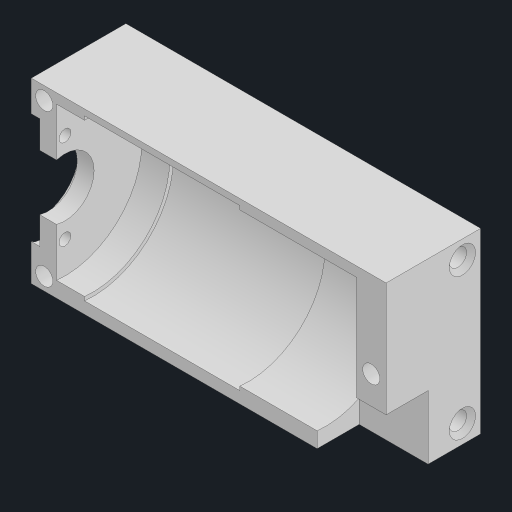
# Autodesk Inventor part: right_motor_holder
Saved by Autodesk Inventor 2023 (Build 270158000, 158)
## iProperties
Created: 2024-04-24
Part Number: right_motor_holder
Material: Generic
Document SubType Name: Modeling
Designer: szymo
Density: 1 g/cm^3
Appearance: Default
Author: szymo
Autodesk Inventor part; units mm, degrees
ref_plane "YZ Plane" through (0, 0, 0) normal (1, 0, 0) x (0, 1, 0)
ref_plane "XZ Plane" through (0, 0, 0) normal (0, 1, 0) x (-1, 0, 0)
ref_plane "XY Plane" through (0, 0, 0) normal (0, 0, 1) x (1, 0, 0)
ref_plane "Work Plane1" through (-42.7, -68.375, 15.375) normal (1, 0, 0) x (0, -1, 0)
sketch "Sketch1" plane through (-42.7, -68.375, 15.375) normal (1, 0, 0) x (0, -1, 0)
  circle A0 centre (0, 0) radius 14.375 projected
  circle A1 centre (0, 0) radius 13.7 projected
  line L0 (90.625, 18.375) -> (-15.375, 18.375) projected
  line L1 (-15.375, 18.375) -> (-15.375, 15.375) projected
  line L2 (90.625, 15.375) -> (-15.375, 15.375) projected
  line L3 (90.625, 18.375) -> (90.625, 15.375) projected
  line L4 (-15.375, 15.375) -> (16.375, 15.375)
  line L5 (16.375, 15.375) -> (16.375, -1.5)
  line L6 (16.375, -1.5) -> (-15.375, -1.5)
  line L7 (-15.375, -1.5) -> (-15.375, 15.375)
  circle A2 centre (0, 0) radius 13.9
  point P0 (-68.375, 15.375)
  point P1 (14.375, 0)
  point P2 (-13.6176, -1.5)
  point P3 (13.6176, -1.5)
  point P4 (16.375, 15.375)
  dimension "d1" = 2
  dimension "d2" = 1.5
  dimension "d3" = 0.2
  constraints: 8 end point, 2 parallel, 1 centre point, 1 horizontal, 1 horizontal alignment, 1 perpendicular, 2 other
  measures "d1" distance from line of L5 point (14.375, 0)
  measures "d2" distance from line of L6 point (14.375, 0)
  measures "d3" radial gap between concentric circles of A1 A2
extrude "Extrusion1" add sketch "Sketch1" along normal blind 9.5 contours A0 L6 A2 | A0 L6 L7 L2 L5 | A2 L6 A1 picked at (14.0681, 1.1841) picked at (-2.3687, 13.4988)
ref_plane "Work Plane2" through (-37.7, -68.375, 15.375) normal (1, 0, 0) x (0, -1, 0)
sketch "Sketch2" plane through (-37.7, -68.375, 15.375) normal (1, 0, 0) x (0, -1, 0)
  arc A0 (13.6176, -1.5) -> (-13.6176, -1.5) centre (0, 0) ccw projected
  line L0 (13.6176, -1.5) -> (16.375, -1.5) projected
  line L1 (16.375, -1.5) -> (16.375, 15.375) projected
  line L2 (16.375, 15.375) -> (-15.375, 15.375) projected
  line L3 (-15.375, 15.375) -> (-15.375, -1.5) projected
  line L4 (-15.375, -1.5) -> (-13.6176, -1.5) projected
  circle A1 centre (8, 0) radius 1.0564 projected
  circle A2 centre (-8, 0) radius 1.0564 projected
  circle A3 centre (0, 0) radius 5 projected
  circle A4 centre (0, 0) radius 13.7 projected
  circle A5 centre (0, 0) radius 5.2
  arc A6 (13.6176, -1.5) -> (-13.6176, -1.5) centre (0, 0) ccw projected
  line L5 (13.6176, -1.5) -> (-13.6176, -1.5)
  point P0 (-68.375, 15.375)
  point P1 (4.979, -1.5)
  point P2 (-4.979, -1.5)
  dimension "d6" = 0.2
  constraints: 2 end point, 1 centre point, 1 collinear
  measures "d6" radial gap between concentric circles of A3 A5
extrude "Extrusion2" add sketch "Sketch2" along normal blind 3 contours L5 A5 A0
sketch "Sketch3" plane through (-34.7, -68.375, 15.375) normal (1, 0, 0) x (0, 0, -1)
  arc A0 (-1.5, -13.6176) -> (-1.5, 13.6176) centre (0, 0) ccw projected
  line L0 (-1.5, 13.6176) -> (-1.5, 4.979) projected
  arc A1 (-1.5, -4.979) -> (-1.5, 4.979) centre (0, 0) ccw projected
  line L1 (-1.5, -4.979) -> (-1.5, -13.6176) projected
  circle A2 centre (0, -8) radius 1.0564 projected
  circle A3 centre (0, 8) radius 1.0564 projected
  arc A4 (0.512, -3.83) -> (1.6707, -5.5993) centre (4.9979, -2.1562) ccw projected
  arc A5 (1.6707, -5.5993) -> (2.5261, -5.269) centre (0, 0) ccw projected
  arc A6 (2.5261, -5.269) -> (2.195, -3.1802) centre (-2.2517, -4.9556) ccw projected
  arc A7 (2.195, -3.1802) -> (2.6654, -2.7976) centre (0, 0) ccw projected
  arc A8 (2.6654, -2.7976) -> (4.6428, -3.548) centre (5.3108, 1.1933) ccw projected
  arc A9 (4.6428, -3.548) -> (5.1407, -2.778) centre (0, 0) ccw projected
  arc A10 (5.1407, -2.778) -> (3.645, -1.2826) centre (1.0912, -5.3327) ccw projected
  arc A11 (3.645, -1.2826) -> (3.8008, -0.6966) centre (0, 0) ccw projected
  arc A12 (3.8008, -0.6966) -> (5.8416, -0.1414) centre (3.5951, 4.087) ccw projected
  arc A13 (5.8416, -0.1414) -> (5.7918, 0.7742) centre (0, 0) ccw projected
  arc A14 (5.7918, 0.7742) -> (3.7028, 1.1048) centre (4.0173, -3.6729) ccw projected
  arc A15 (3.7028, 1.1048) -> (3.4844, 1.6705) centre (0, 0) ccw projected
  arc A16 (3.4844, 1.6705) -> (4.809, 3.3192) centre (0.5063, 5.4196) ccw projected
  arc A17 (4.809, 3.3192) -> (4.2306, 4.0306) centre (0, 0) ccw projected
  arc A18 (4.2306, 4.0306) -> (2.3462, 3.0703) centre (5.4089, -0.6101) ccw projected
  arc A19 (2.3462, 3.0703) -> (1.8371, 3.3995) centre (0, 0) ccw projected
  arc A20 (1.8371, 3.3995) -> (1.9396, 5.512) centre (-2.776, 4.6821) ccw projected
  arc A21 (1.9396, 5.512) -> (1.0535, 5.7475) centre (0, 0) ccw projected
  arc A22 (1.0535, 5.7475) -> (0.0935, 3.863) centre (4.7345, 2.6857) ccw projected
  arc A23 (0.0935, 3.863) -> (-0.512, 3.83) centre (0, 0) ccw projected
  arc A24 (-0.512, 3.83) -> (-1.6707, 5.5993) centre (-4.9979, 2.1562) ccw projected
  arc A25 (-1.6707, 5.5993) -> (-2.5261, 5.269) centre (0, 0) ccw projected
  arc A26 (-2.5261, 5.269) -> (-2.195, 3.1802) centre (2.2517, 4.9556) ccw projected
  arc A27 (-2.195, 3.1802) -> (-2.6654, 2.7976) centre (0, 0) ccw projected
  arc A28 (-2.6654, 2.7976) -> (-4.6428, 3.548) centre (-5.3108, -1.1933) ccw projected
  arc A29 (-4.6428, 3.548) -> (-5.1407, 2.778) centre (0, 0) ccw projected
  arc A30 (-5.1407, 2.778) -> (-3.645, 1.2826) centre (-1.0912, 5.3327) ccw projected
  arc A31 (-3.645, 1.2826) -> (-3.8008, 0.6966) centre (0, 0) ccw projected
  arc A32 (-3.8008, 0.6966) -> (-5.8416, 0.1414) centre (-3.5951, -4.087) ccw projected
  arc A33 (-5.8416, 0.1414) -> (-5.7918, -0.7742) centre (0, 0) ccw projected
  arc A34 (-5.7918, -0.7742) -> (-3.7028, -1.1048) centre (-4.0173, 3.6729) ccw projected
  arc A35 (-3.7028, -1.1048) -> (-3.4844, -1.6705) centre (0, 0) ccw projected
  arc A36 (-3.4844, -1.6705) -> (-4.809, -3.3192) centre (-0.5063, -5.4196) ccw projected
  arc A37 (-4.809, -3.3192) -> (-4.2306, -4.0306) centre (0, 0) ccw projected
  arc A38 (-4.2306, -4.0306) -> (-2.3462, -3.0703) centre (-5.4089, 0.6101) ccw projected
  arc A39 (-2.3462, -3.0703) -> (-1.8371, -3.3995) centre (0, 0) ccw projected
  arc A40 (-1.8371, -3.3995) -> (-1.9396, -5.512) centre (2.776, -4.6821) ccw projected
  arc A41 (-1.9396, -5.512) -> (-1.0535, -5.7475) centre (0, 0) ccw projected
  arc A42 (-1.0535, -5.7475) -> (-0.0935, -3.863) centre (-4.7345, -2.6857) ccw projected
  arc A43 (-0.0935, -3.863) -> (0.512, -3.83) centre (0, 0) ccw projected
  circle A44 centre (0, 0) radius 7
  arc A45 (-1.5, -13.6176) -> (-1.5, 13.6176) centre (0, 0) ccw projected
  line L2 (-1.5, -13.6176) -> (-1.5, -16.375) projected
  line L3 (-1.5, -16.375) -> (15.375, -16.375) projected
  line L4 (15.375, -16.375) -> (15.375, 15.375) projected
  line L5 (15.375, 15.375) -> (-1.5, 15.375) projected
  line L6 (-1.5, 15.375) -> (-1.5, 13.6176) projected
  circle A46 centre (0, -8) radius 2.4
  circle A47 centre (0, 8) radius 2.4
  circle A48 centre (0, 0) radius 5.8433
  point P0 (15.375, 68.375)
  point P1 (2.019, 6.7025)
  point P2 (2.019, -6.7025)
  point P3 (-1.5, -9.8735)
  point P4 (-1.5, 9.8735)
  dimension "d9" = 14
  dimension "d10" = 4.8
  dimension "d11" = 4.8
  constraints: 4 centre point, 4 coincident, 1 concentric
  measures "d9" diameter of A44
  measures "d10" diameter of A46
  measures "d11" diameter of A47
extrude "Extrusion3" add sketch "Sketch3" along normal up to surface (1.5 mm away) contours L1 A46 A44 A47 L0 A0
sketch "Sketch4" plane through (-42.7, -84.75, 16.875) normal (0, 0, 1) x (1, 0, 0)
  line L0 (0, 2.7574) -> (0, 0) projected
  line L1 (0, 0) -> (9.5, 0) projected
  line L2 (9.5, 0) -> (9.5, 6.5015) projected
  line L3 (8, 6.5015) -> (9.5, 6.5015) projected
  line L4 (8, 11.396) -> (8, 6.5015) projected
  line L5 (5, 11.396) -> (8, 11.396) projected
  line L6 (5, 11.396) -> (5, 2.7574) projected
  line L7 (0, 2.7574) -> (5, 2.7574) projected
  line L8 (0, 31.75) -> (0, 29.9926) projected
  line L9 (0, 29.9926) -> (5, 29.9926) projected
  line L10 (5, 29.9926) -> (5, 21.354) projected
  line L11 (5, 21.354) -> (8, 21.354) projected
  line L12 (8, 26.2485) -> (8, 21.354) projected
  line L13 (8, 26.2485) -> (9.5, 26.2485) projected
  line L14 (9.5, 31.75) -> (9.5, 26.2485) projected
  line L15 (0, 31.75) -> (9.5, 31.75) projected
  circle A0 centre (7.2, 2.3) radius 2.5
  circle A1 centre (7.2, 29.45) radius 2.5
  point P0 (42.7, 84.75)
  dimension "d14" = 5
  dimension "d15" = 5
  dimension "d16" = 2.3
  dimension "d17" = 2.3
  dimension "d18" = 2.3
  dimension "d19" = 2.3
  constraints: 2 centre point, 2 coincident
  measures "d14" diameter of A0
  measures "d15" diameter of A1
  measures "d16" distance from line of A1.centre L14
  measures "d17" distance from line of A1.centre L15
  measures "d18" distance from line of L1 A0.centre
  measures "d19" distance from line of L2 A0.centre
hole "Hole1" at (-35.5, -82.45, 16.875) at (-35.5, -55.3, 16.875) direction (0, 0, -1) diameter 3.1 end through all clearance for "Countersunk Flat Head Screw ISO 2009/7046" size "M2.5" standard "ISO"
sketch "Sketch5" plane through (-42.7, -68.375, 15.375) normal (-1, 0, 0) x (0, 0, 1)
  circle A0 centre (0, 0) radius 14.375 projected
  arc A1 (1.5, 13.6176) -> (1.5, -13.6176) centre (0, 0) ccw projected
  line L0 (1.5, 15.375) -> (1.5, 13.6176) projected
  line L1 (-15.375, 15.375) -> (1.5, 15.375) projected
  line L2 (-15.375, -16.375) -> (-15.375, 15.375) projected
  line L3 (1.5, -16.375) -> (-15.375, -16.375) projected
  line L4 (1.5, -13.6176) -> (1.5, -16.375) projected
  point P0 (-15.375, 68.375)
  point P1 (1.5, -14.2965)
  point P2 (1.5, 14.2965)
ref_plane "Work Plane3" through (-70.4, -82.75, 1) normal (-1, 0, 0) x (0, 0, 1)
extrude "Extrusion4" add sketch "Sketch5" along normal up to surface (27.7 mm away) contours A0 L4 L3 L2 L1 L0
sketch "Sketch6" plane through (-70.4, -68.375, 15.375) normal (-1, 0, 0) x (0, 0, 1)
  line L0 (-15.375, 15.375) -> (1.5, 15.375) projected
  line L1 (-15.375, -16.375) -> (-15.375, 15.375) projected
  line L2 (1.5, -16.375) -> (-15.375, -16.375) projected
  line L3 (1.5, -14.2965) -> (1.5, -16.375) projected
  arc A0 (1.5, 14.2965) -> (1.5, -14.2965) centre (0, 0) ccw projected
  line L4 (1.5, 15.375) -> (1.5, 14.2965) projected
  circle A1 centre (0, 0) radius 13.7 projected
  line L5 (-15.375, 15.375) -> (1.5, 15.375)
  line L6 (1.5, 15.375) -> (1.5, -16.375)
  line L7 (1.5, -16.375) -> (-15.375, -16.375)
  line L8 (-15.375, -16.375) -> (-15.375, 15.375)
  point P0 (-15.375, 68.375)
  point P1 (1.5, 14.2965)
  point P2 (1.5, -14.2965)
  point P3 (1.5, -13.6176)
  point P4 (1.5, 13.6176)
  constraints: 8 end point, 2 parallel, 1 horizontal, 1 perpendicular
ref_plane "Work Plane4" through (-84.2, -82.075, 1.675) normal (-1, 0, 0) x (0, 0, 1)
extrude "Extrusion5" add sketch "Sketch6" along normal up to surface (13.8 mm away) contours L0 L4 A0 L3 L2 L1 | L6 A1 A0
sketch "Sketch7" plane through (-84.2, -68.375, 15.375) normal (-1, 0, 0) x (0, 0, 1)
  line L0 (1.5, 15.375) -> (1.5, 13.6176) projected
  line L1 (-15.375, 15.375) -> (1.5, 15.375) projected
  line L2 (-15.375, -16.375) -> (-15.375, 15.375) projected
  line L3 (1.5, -16.375) -> (-15.375, -16.375) projected
  line L4 (1.5, -13.6176) -> (1.5, -16.375) projected
  arc A0 (1.5, 13.6176) -> (1.5, -13.6176) centre (0, 0) ccw projected
  line L5 (-1.5, 11) -> (-1.5, 11.5) projected
  line L6 (-1.5, 11.5) -> (1.5, 11.5) projected
  line L7 (1.5, 11.5) -> (1.5, 11) projected
  line L8 (1.5, 11) -> (-1.5, 11) projected
  line L9 (1.5, -11.5) -> (1.5, -12) projected
  line L10 (1.5, -12) -> (-1.5, -12) projected
  line L11 (-1.5, -12) -> (-1.5, -11.5) projected
  line L12 (-1.5, -11.5) -> (1.5, -11.5) projected
  circle A1 centre (0, 0) radius 5 projected
  circle A2 centre (0, 0) radius 13.7 projected
  line L13 (-15.375, 15.375) -> (1.5, 15.375) projected
  line L14 (-15.375, -16.375) -> (-15.375, 15.375) projected
  line L15 (-6, 15.375) -> (-15.375, 15.375)
  line L16 (-15.375, 15.375) -> (-15.375, -16.375)
  line L17 (-15.375, -16.375) -> (-6, -16.375)
  line L18 (-6, -16.375) -> (-6, 15.375)
  point P0 (-15.375, 68.375)
  point P1 (-5, 0)
  point P2 (-6, 15.375)
  point P3 (-6, -16.375)
  point P4 (-6, 12.3162)
  dimension "d31" = 1
  constraints: 8 end point, 2 parallel, 1 horizontal, 1 horizontal alignment, 1 perpendicular, 1 point on line, 2 other
  measures "d31" distance from line of L18 point (-5, 0)
ref_plane "Work Plane5" through (-96.5, -125.8889, 0) normal (1, 0, 0) x (0, 1, 0)
extrude "Extrusion6" add sketch "Sketch7" along normal up to surface (12.3 mm away) contours L0 A0 L18 L1 | L18 A0 L3 L2 L1 | L18 A0
sketch "Sketch8" plane through (-84.2, -80.6912, 9.375) normal (0, 0, 1) x (1, 0, 0)
  line L0 (-12.3, -4.0588) -> (-12.3, 24.6325) projected
  line L1 (0, -4.0588) -> (-12.3, -4.0588) projected
  line L2 (0, 0) -> (0, -4.0588) projected
  line L3 (0, 0) -> (0, 24.6325) projected
  line L4 (0, 24.6325) -> (-12.3, 24.6325) projected
  circle A0 centre (48.7, 25.3912) radius 1.55 projected
  line L5 (41.5, 26.6128) -> (41.5, 25.9339) projected
  line L6 (41.5, 25.9339) -> (46.5, 25.9339) projected
  line L7 (46.5, 25.9339) -> (46.5, 17.2952) projected
  line L8 (46.5, 17.2952) -> (49.5, 17.2952) projected
  line L9 (49.5, 22.1897) -> (49.5, 17.2952) projected
  line L10 (49.5, 22.1897) -> (51, 22.1897) projected
  line L11 (51, 27.6912) -> (51, 22.1897) projected
  line L12 (51, 27.6912) -> (-12.3, 27.6912) projected
  line L13 (-12.3, 25.9339) -> (-12.3, 27.6912) projected
  line L14 (13.8, 25.9339) -> (-12.3, 25.9339) projected
  line L15 (13.8, 25.9339) -> (13.8, 26.6128) projected
  line L16 (41.5, 26.6128) -> (13.8, 26.6128) projected
  line L17 (0, 24.6325) -> (0, 0) projected
  line L18 (0, 0) -> (0, -1.3014) projected
  line L19 (13.8, -1.3014) -> (0, -1.3014) projected
  line L20 (13.8, -1.3014) -> (13.8, 25.9339) projected
  line L21 (13.8, 25.9339) -> (-12.3, 25.9339) projected
  line L22 (-12.3, 24.6325) -> (-12.3, 25.9339) projected
  line L23 (0, 24.6325) -> (-12.3, 24.6325) projected
  line L24 (0, 23.8162) -> (0, 23.3162) projected
  line L25 (0, 23.8162) -> (-6, 23.8162) projected
  line L26 (-6, 23.3162) -> (-6, 23.8162) projected
  line L27 (0, 23.3162) -> (-6, 23.3162) projected
  line L28 (0, 0.8162) -> (0, 0.3162) projected
  line L29 (0, 0.8162) -> (-6, 0.8162) projected
  line L30 (-6, 0.3162) -> (-6, 0.8162) projected
  line L31 (0, 0.3162) -> (-6, 0.3162) projected
  line L32 (-12.3, 27.6912) -> (-12.3, -4.0588) projected
  line L33 (-12.3, -4.0588) -> (51, -4.0588) projected
  line L34 (-12.3, 27.6912) -> (-7, 27.6912)
  line L35 (-7, 27.6912) -> (-7, -4.0588)
  line L36 (-7, -4.0588) -> (-12.3, -4.0588)
  line L37 (-12.3, -4.0588) -> (-12.3, 27.6912)
  line L38 (-7, -4.0588) -> (-12.3, -4.0588)
  line L39 (-12.3, -4.0588) -> (-12.3, 7.3162)
  line L40 (-12.3, 7.3162) -> (-7, 7.3162)
  line L41 (-7, 7.3162) -> (-7, -4.0588)
  line L42 (0, 7.3162) -> (-4, 7.3162)
  point P0 (84.2, 80.6912)
  point P1 (-7, -4.0588)
  point P2 (-7, 27.6912)
  point P3 (-12.3, 25.9339)
  point P4 (-12.3, 7.3162)
  point P5 (-7, 7.3162)
  dimension "d34" = 1
  constraints: 18 end point, 4 parallel, 3 horizontal, 2 perpendicular, 2 point on line, 1 collinear, 2 other
  measures "d34" distance between parallel lines of L26 L35
extrude "Extrusion7" add sketch "Sketch8" along normal up to surface (7.5 mm away) contours L0 L4 L35 L40 | L22 L14 L35 L4 | L13 L12 L35 L14
sketch "Sketch9" plane through (-37.7, -63.396, 16.875) normal (0, 0, 1) x (1, 0, 0)
  line L0 (-46.5, 0.021) -> (-50.5, 0.021)
  line L1 (-50.5, 0.021) -> (-50.5, -9.979) projected
  line L2 (-46.5, -9.979) -> (-50.5, -9.979)
  line L3 (-58.8, 10.396) -> (-58.8, -21.354) projected
  line L4 (-50.5, -9.979) -> (-58.8, -9.979)
  line L5 (-58.8, -9.979) -> (-58.8, 0.021)
  line L6 (-58.8, 0.021) -> (-50.5, 0.021)
  line L7 (-50.5, 0.021) -> (-50.5, -9.979)
  line L8 (-53.5, 7.3373) -> (-53.5, -9.979) projected
  line L9 (-53.5, 0.021) -> (-53.5, -9.979)
  line L10 (-53.5, 0.021) -> (-58.8, -9.979)
  line L11 (-53.5, -9.979) -> (-58.8, 0.021)
  point P0 (37.7, 63.396)
  point P1 (-56.15, -4.979)
  constraints: 18 end point, 3 horizontal, 3 point on line, 2 parallel, 2 perpendicular, 1 collinear, 1 midpoint, 3 other
hole "Hole2" at (-93.85, -68.375, 16.875) direction (0, 0, -1) diameter 3.1 end through all clearance for "Countersunk Flat Head Screw ISO 2009/7046" size "M2.5" standard "ISO"
sketch "Sketch10" plane through (-96.5, -84.75, 0) normal (-1, 0, 0) x (0, 0, 1)
  circle A0 centre (15.375, 16.375) radius 14.375 projected
  line L0 (16.875, 31.75) -> (0, 31.75) projected
  line L1 (0, 31.75) -> (0, 0) projected
  line L2 (0, 0) -> (9.375, 0) projected
  line L3 (9.375, 0) -> (9.375, 11.375) projected
  line L4 (9.375, 11.375) -> (16.875, 11.375) projected
  line L5 (16.875, 11.375) -> (16.875, 31.75) projected
  line L6 (0, 31.75) -> (16.875, 31.75) projected
  line L7 (0, 31.75) -> (6.5, 31.75)
  line L8 (6.5, 31.75) -> (6.5, 25.25)
  line L9 (6.5, 25.25) -> (0, 25.25)
  line L10 (0, 25.25) -> (0, 31.75)
  line L11 (0, 0) -> (0, 31.75) projected
  line L12 (0, 0) -> (6.5, 0)
  line L13 (6.5, 0) -> (6.5, 6.5)
  line L14 (6.5, 6.5) -> (0, 6.5)
  line L15 (0, 6.5) -> (0, 0)
  line L16 (6.5, 31.75) -> (0, 25.25)
  line L17 (6.5, 25.25) -> (0, 31.75)
  line L18 (0, 0) -> (6.5, 6.5)
  line L19 (6.5, 0) -> (0, 6.5)
  circle A1 centre (3.25, 28.5) radius 1.8
  circle A2 centre (3.25, 3.25) radius 1.8
  point P0 (0, 84.75)
  dimension "d44" = 6.5
  dimension "d45" = 6.5
  dimension "d46" = 6.5
  dimension "d47" = 6.5
  dimension "d48" = 3.6
  dimension "d49" = 3.6
  constraints: 24 end point, 4 parallel, 2 centre point, 2 coincident, 2 horizontal, 2 midpoint, 2 perpendicular
  measures "d44" distance of L8.end L9.end
  measures "d45" distance of L7.end L8.end
  measures "d46" distance of L14.end L13.end
  measures "d47" distance of L13.end L12.end
  measures "d48" diameter of A1
  measures "d49" diameter of A2
hole "Hole3" at (-96.5, -56.25, 3.25) at (-96.5, -81.5, 3.25) direction (1, 0, 0) diameter 3.1 depth 20 clearance for "Countersunk Flat Head Screw ISO 2009/7046" size "M3" standard "ISO"
chamfer "Chamfer1" distance 0.8 angle 45 2 edges at (-96.5, -56.25, 1.7) (-96.5, -81.5, 1.7)
mirror "Mirror1" about plane through (0, 0, 0) normal (1, 0, 0) remove original yes
equation "\"d44\" = d45"
equation "\"d46\" = d45"
equation "\"d47\" = d45"
body "Solid1"
